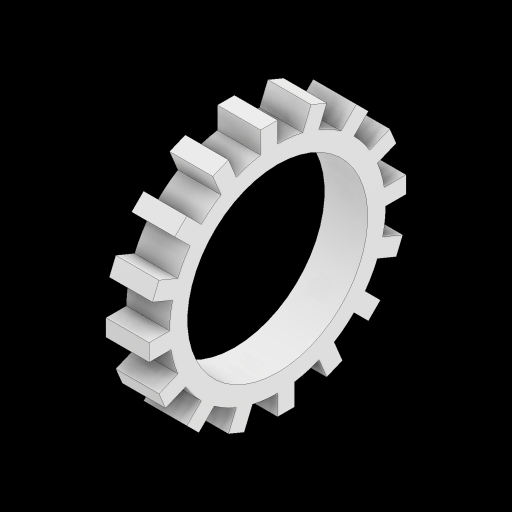
# Autodesk Inventor part: wedge holder
Saved by Autodesk Inventor 2023 (Build 270158000, 158)
## iProperties
Created: 2023-07-14
Part Number: wedge holder
Material: ABS Plastic
Document SubType Name: Modeling
Designer: pif12
Density: 1.06 g/cm^3
Appearance: Smooth - White
Author: pif12
Autodesk Inventor part; units mm, degrees
ref_plane "YZ Plane" through (0, 0, 0) normal (1, 0, 0) x (0, 1, 0)
ref_plane "XZ Plane" through (0, 0, 0) normal (0, 1, 0) x (-1, 0, 0)
ref_plane "XY Plane" through (0, 0, 0) normal (0, 0, 1) x (1, 0, 0)
sketch "Sketch1" plane through (0, 0, 0) normal (1, 0, 0) x (0, 1, 0)
  circle A0 centre (0, 0) radius 13.25
  circle A1 centre (0, 0) radius 15.875
  line L0 (15.875, 0) -> (18.875, 0)
  line L1 (18.875, 0) -> (18.875, 2.5)
  line L2 (18.875, 2.5) -> (15.6769, 2.5)
  line L3 (17.4382, 7.2231) -> (16.4815, 9.5328)
  line L4 (16.4815, 9.5328) -> (13.5269, 8.309)
  line L5 (14.6666, 6.0751) -> (17.4382, 7.2231)
  line L6 (13.3466, 13.3466) -> (11.5789, 15.1144)
  line L7 (11.5789, 15.1144) -> (9.3175, 12.853)
  line L8 (11.2253, 11.2253) -> (13.3466, 13.3466)
  line L9 (7.2231, 17.4382) -> (4.9135, 18.3949)
  line L10 (4.9135, 18.3949) -> (3.6896, 15.4403)
  line L11 (6.0751, 14.6666) -> (7.2231, 17.4382)
  line L12 (0, 18.875) -> (-2.5, 18.875)
  line L13 (-2.5, 18.875) -> (-2.5, 15.6769)
  line L14 (0, 15.875) -> (0, 18.875)
  line L15 (-7.2231, 17.4382) -> (-9.5328, 16.4815)
  line L16 (-9.5328, 16.4815) -> (-8.309, 13.5269)
  line L17 (-6.0751, 14.6666) -> (-7.2231, 17.4382)
  line L18 (-13.3466, 13.3466) -> (-15.1144, 11.5789)
  line L19 (-15.1144, 11.5789) -> (-12.853, 9.3175)
  line L20 (-11.2253, 11.2253) -> (-13.3466, 13.3466)
  line L21 (-17.4382, 7.2231) -> (-18.3949, 4.9135)
  line L22 (-18.3949, 4.9135) -> (-15.4403, 3.6896)
  line L23 (-14.6666, 6.0751) -> (-17.4382, 7.2231)
  line L24 (-18.875, 0) -> (-18.875, -2.5)
  line L25 (-18.875, -2.5) -> (-15.6769, -2.5)
  line L26 (-15.875, 0) -> (-18.875, 0)
  line L27 (-17.4382, -7.2231) -> (-16.4815, -9.5328)
  line L28 (-16.4815, -9.5328) -> (-13.5269, -8.309)
  line L29 (-14.6666, -6.0751) -> (-17.4382, -7.2231)
  line L30 (-13.3466, -13.3466) -> (-11.5789, -15.1144)
  line L31 (-11.5789, -15.1144) -> (-9.3175, -12.853)
  line L32 (-11.2253, -11.2253) -> (-13.3466, -13.3466)
  line L33 (-7.2231, -17.4382) -> (-4.9135, -18.3949)
  line L34 (-4.9135, -18.3949) -> (-3.6896, -15.4403)
  line L35 (-6.0751, -14.6666) -> (-7.2231, -17.4382)
  line L36 (0, -18.875) -> (2.5, -18.875)
  line L37 (2.5, -18.875) -> (2.5, -15.6769)
  line L38 (0, -15.875) -> (0, -18.875)
  line L39 (7.2231, -17.4382) -> (9.5328, -16.4815)
  line L40 (9.5328, -16.4815) -> (8.309, -13.5269)
  line L41 (6.0751, -14.6666) -> (7.2231, -17.4382)
  line L42 (13.3466, -13.3466) -> (15.1144, -11.5789)
  line L43 (15.1144, -11.5789) -> (12.853, -9.3175)
  line L44 (11.2253, -11.2253) -> (13.3466, -13.3466)
  line L45 (17.4382, -7.2231) -> (18.3949, -4.9135)
  line L46 (18.3949, -4.9135) -> (15.4403, -3.6896)
  line L47 (14.6666, -6.0751) -> (17.4382, -7.2231)
  dimension "d1" = 31.75
  dimension "d0" = 26.5
  dimension "d3" = 3
  dimension "d4" = 2.5
  dimension "d7" = 360
  constraints: 96 end point, 2 coincident, 2 perpendicular, 1 centre point, 1 horizontal, 117 other
  measures "d0" diameter of A0
  measures "d3" distance of L0.start L0.end
  measures "d4" distance of L0.end L1.end
extrude "Extrusion1" add sketch "Sketch1" along normal blind 6.35
body "Solid1"
